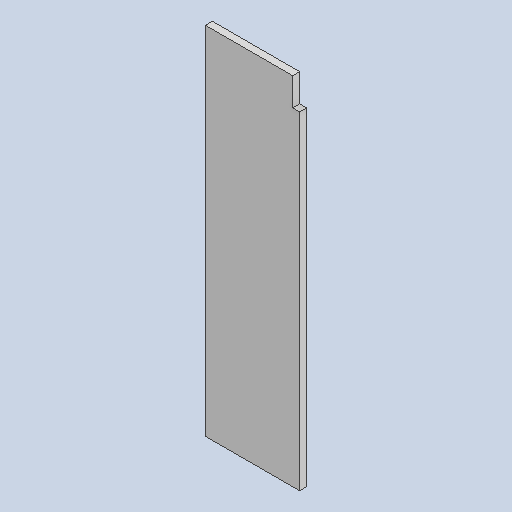
# Autodesk Inventor part: DMF2.0 01 42 Gear way 2
Saved by Autodesk Inventor 2025 (Build 290162010, 162A)
## iProperties
Created: 2024-04-30
Part Number: DMF2.0 01 42 Gear way 2
Material: Generic
Document SubType Name: Sheet Metal
Designer: admin
Stock Number: Барабан_Сектор_Усилителя
Density: 1 g/cm^3
Sheet Metal Rule: Default
Sheet Metal Width: 0,000 mm
Sheet Metal Length: 0,000 mm
Sheet Metal Area: 0,000 mm^2
Appearance: Default
Author: pokla
Autodesk Inventor part; units mm, degrees
ref_plane "YZ Plane" through (0, 0, 0) normal (1, 0, 0) x (0, 1, 0)
ref_plane "XZ Plane" through (0, 0, 0) normal (0, 1, 0) x (-1, 0, 0)
ref_plane "XY Plane" through (0, 0, 0) normal (0, 0, 1) x (1, 0, 0)
sketch "Sketch1" plane through (0, 0, 0) normal (0, 0, 1) x (1, 0, 0)
  line L0 (-13.5, 102) -> (13.5, 102)
  line L1 (13.5, 102) -> (13.5, 0)
  line L2 (13.5, 0) -> (-13.5, 0)
  line L3 (-13.5, 0) -> (-13.5, 102)
  line L4 (13.5, 94) -> (-13.5, 94)
  line L5 (11.5, 94) -> (11.5, 102)
  point P0 (0, 0)
  point P1 (0, 0)
  point P2 (0, 0)
  point P3 (0, 0)
  point P4 (0, 0)
  dimension "d27" = 27
  dimension "d29" = 102
  dimension "d30" = 2
  dimension "d31" = 8
  measures "d27" distance of L1.end L2.end
  measures "d29" distance between parallel lines of L2 L0
  measures "d30" distance between parallel lines of L1 L5
  measures "d31" distance between parallel lines of L4 L0
extrude "Plate1" add sketch "Sketch1" along normal mid plane 2 contours L0 L5 L4 L3 | L4 L1 L2 L3
equation "\"d29\" = 0.5 * Шстр_диам_внутр - 0.5 * Колесо_диам_3 - 2 * Thickness"
equation "\"d30\" = Thickness"
equation "\"d31\" = 0.5 * Шстр_диам_внутр - 0.5 * Колесо_диам_2 - Thickness"
equation "\"d15\" = Thickness"
equation "\"BendRadius\" = Thickness"
equation "\"BendReliefWidth\" = Thickness"
equation "\"BendReliefDepth\" = 0.5 * Thickness"
equation "\"CornerReliefSize\" = 4 * Thickness"
equation "\"MinimumRemnant\" = 2 * Thickness"
equation "\"TransitionRadius\" = BendRadius"
equation "\"JacobiRadiusSize\" = BendRadius"
equation "\"GapSize\" = Thickness"
equation "\"Шстр_диам_внутр\" = 720"
equation "\"Колесо_диам_3\" = 508"
equation "\"Thickness\" = 2"
equation "\"Колесо_диам_2\" = 700"
body "Solid1"
